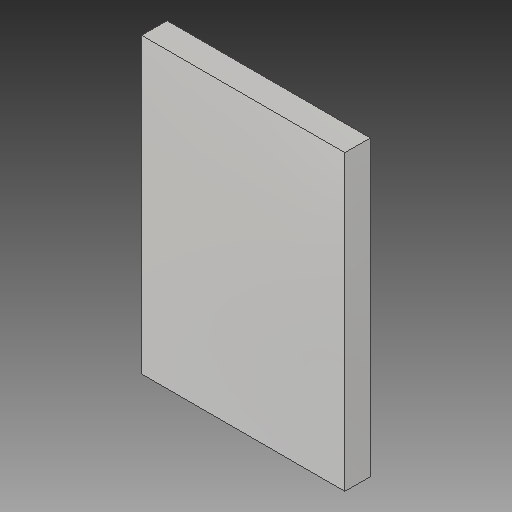
# Autodesk Inventor part: suporte_boca_soprador
Saved by Autodesk Inventor 2018 (Build 220112000, 112)
## iProperties
Created: 2018-05-10
Part Number: suporte_boca_soprador
Material: Alumínio-6061-AHC
Document SubType Name: Modeling
Designer: Georgines
Density: 2.7 g/cm^3
Appearance: Alumínio - Escuro
Mass: 216.13 g
Surface Area: 203.204 cm^2
Volume: 80.0481 cm^3
Author: Georgines
Autodesk Inventor part; units mm, degrees
ref_plane "YZ Plane" through (0, 0, 0) normal (1, 0, 0) x (0, 1, 0)
ref_plane "XZ Plane" through (0, 0, 0) normal (0, 1, 0) x (-1, 0, 0)
ref_plane "XY Plane" through (0, 0, 0) normal (0, 0, 1) x (1, 0, 0)
sketch "Esboço1" plane through (0, 0, 0) normal (0, 0, 1) x (1, 0, 0)
  line L0 (-2, 75.533) -> (-2, -34.467)
  line L1 (74.2, -34.467) -> (74.2, 75.533)
  line L2 (-2, -34.467) -> (74.2, -34.467)
  line L3 (-2, 75.533) -> (74.2, 75.533)
  line L4 (36.1, -19.227) -> (36.1, -34.467) construction
  dimension "d48" = 76.2
  dimension "d49" = 110
  constraints: 10 end point, 2 perpendicular, 1 midpoint, 1 parallel
  measures "d48" distance of L0.start L1.end
  measures "d49" distance of L0.start L0.end
extrude "Extrusão1" add sketch "Esboço1" along normal blind 9.55
